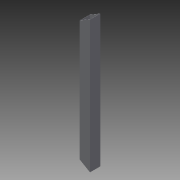
# Autodesk Inventor part: Square_30degree
Saved by Autodesk Inventor 2015 SP1 (Build 190203100, 203)
## iProperties
Created: 2016-02-02
Part Number: Square_30degree
Material: Generic
Document SubType Name: Modeling
Designer: guillemd
Density: 1 g/cm^3
Appearance: Default
Author: guillemd
Autodesk Inventor part; units mm, degrees
ref_plane "YZ Plane" through (0, 0, 0) normal (1, 0, 0) x (0, 1, 0)
ref_plane "XZ Plane" through (0, 0, 0) normal (0, 1, 0) x (-1, 0, 0)
ref_plane "XY Plane" through (0, 0, 0) normal (0, 0, 1) x (1, 0, 0)
sketch "Sketch1" plane through (0, 0, 0) normal (0, 1, 0) x (-1, 0, 0)
  line L0 (25.4, 25.4) -> (-25.4, 25.4)
  line L1 (-25.4, 25.4) -> (-25.4, -25.4)
  line L2 (-25.4, -25.4) -> (25.4, -25.4)
  line L3 (25.4, -25.4) -> (25.4, 25.4)
  line L4 (-27.5082, 27.5082) -> (27.5082, 27.5082)
  line L5 (27.5082, 27.5082) -> (27.5082, -27.5082)
  line L6 (27.5082, -27.5082) -> (-27.5082, -27.5082)
  line L7 (-27.5082, -27.5082) -> (-27.5082, 27.5082)
  point P0 (0, 0)
  point P1 (25.4, 0)
  point P2 (0, -25.4)
  dimension "d0" = 50.8
  dimension "d1" = 50.8
  dimension "d2" = 2.1082
  constraints: 16 end point, 4 parallel, 2 midpoint, 2 perpendicular, 1 horizontal, 1 horizontal alignment, 1 vertical alignment, 3 other
  measures "d0" distance of L2.end L0.start
  measures "d1" distance of L1.end L2.end
  measures "d2" distance between parallel lines of L0 L4
extrude "Extrusion1" add sketch "Sketch1" along normal blind 711.2
sketch "Sketch2" plane through (-27.5082, 0, 27.5082) normal (0, 0, 1) x (1, 0, 0)
  line L0 (0, 0) -> (55.0164, 0)
  line L1 (55.0164, 0) -> (0, 0) projected
  line L2 (0, 31.7637) -> (55.0164, 0)
  line L3 (0, 0) -> (0, 711.2) projected
  line L4 (0, 31.7637) -> (0, 0)
  line L5 (2.1082, 0) -> (2.1082, 711.2) projected
  line L6 (0, 711.2) -> (55.0164, 711.2)
  line L7 (0, 711.2) -> (55.0164, 711.2) projected
  line L8 (55.0164, 711.2) -> (0, 679.4363)
  line L9 (0, 679.4363) -> (0, 711.2)
  point P0 (27.5082, 0)
  dimension "d5" = 30
  dimension "d6" = 30
  constraints: 12 end point, 2 collinear, 2 parallel, 2 point on line
  measures "d5" angle of L0 L2
  measures "d6" angle of L8 L6
extrude "Extrusion2" cut sketch "Sketch2" against normal through all contours L3 L2 L5 L0 | L5 L2 L0 | L3 L6 L5 L8 | L5 L6 L8
body "Solid1"
